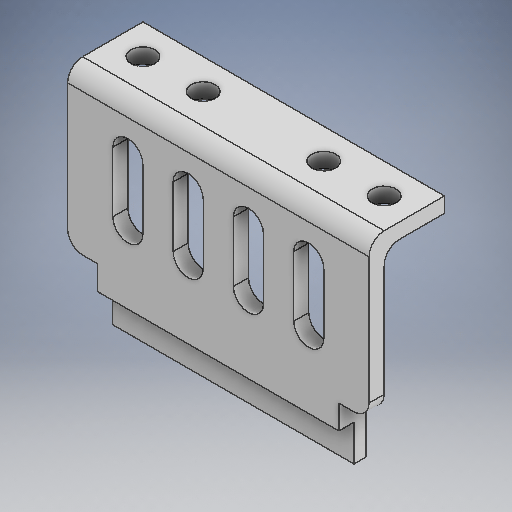
# Autodesk Inventor part: lateral_panel_1
Saved by Autodesk Inventor 2026.1 (Build 301233000, 233)
## iProperties
Created: 2025-12-05
Part Number: lateral_panel_1
Material: Generic
Document SubType Name: Modeling
Designer: emanuel
Density: 1 g/cm^3
Appearance: Default
Author: emanuel
Autodesk Inventor part; units mm, degrees
ref_plane "YZ Plane" through (0, 0, 0) normal (1, 0, 0) x (0, 1, 0)
ref_plane "XZ Plane" through (0, 0, 0) normal (0, 1, 0) x (-1, 0, 0)
ref_plane "XY Plane" through (0, 0, 0) normal (0, 0, 1) x (1, 0, 0)
sketch "Sketch1" plane through (0, 0, 0) normal (1, 0, 0) x (0, 1, 0)
  line L0 (0, 0) -> (30, 0)
  line L1 (30, 0) -> (0, 0)
  line L2 (0, 0) -> (0, -2.5)
  line L3 (0, -2.5) -> (30, -2.5)
  line L4 (30, -2.5) -> (30, 0)
  line L5 (30, -2.5) -> (27.5, -2.5)
  line L6 (27.5, -2.5) -> (27.5, -12.5)
  line L7 (27.5, -12.5) -> (30, -12.5)
  line L8 (30, -12.5) -> (30, -2.5)
  line L9 (0, -2.5) -> (2, -2.5)
  line L10 (2, -2.5) -> (2, -4.5)
  line L11 (2, -4.5) -> (0, -4.5)
  line L12 (0, -4.5) -> (0, -2.5)
  line L13 (0, -2.5) -> (-6, -2.5)
  line L14 (-6, -2.5) -> (-6, -4.5)
  line L15 (-6, -4.5) -> (0, -4.5)
  line L16 (0, -4.5) -> (0, -2.5)
  dimension "d0" = 30
  dimension "d1" = 2.5
  dimension "d2" = 2.5
  dimension "d3" = 10
  dimension "d4" = 2
  dimension "d5" = 2
  dimension "d6" = 6
  constraints: 34 end point, 8 parallel, 5 horizontal, 4 perpendicular, 1 point on line
  measures "d0" distance of L0.start L0.end
  measures "d1" distance of L2.end L1.end
  measures "d2" distance of L7.end L6.end
  measures "d3" distance of L6.end L5.end
  measures "d4" distance of L10.end L11.end
  measures "d5" distance of L9.end L10.end
  measures "d6" distance of L15.end L14.end
extrude "Extrusion1" add sketch "Sketch1" along normal blind 50
sketch "Sketch2" plane through (0, 30, 0) normal (0, 1, 0) x (1, 0, 0)
  line L0 (50, 12.5) -> (50, 0) projected
  line L1 (50, 12.5) -> (45, 12.5)
  line L2 (45, 12.5) -> (45, 7.5)
  line L3 (45, 7.5) -> (50, 7.5)
  line L4 (50, 7.5) -> (50, 12.5)
  line L5 (45, 7.5) -> (35, 7.5)
  line L6 (0, 12.5) -> (50, 12.5) projected
  line L7 (0, 12.5) -> (5, 12.5)
  line L8 (5, 12.5) -> (5, 7.5)
  line L9 (5, 7.5) -> (0, 7.5)
  line L10 (0, 7.5) -> (0, 12.5)
  circle A0 centre (5, 7.5) radius 2
  circle A1 centre (35, 7.5) radius 2
  circle A2 centre (45, 7.5) radius 2
  line L11 (5, 7.5) -> (15, 7.5)
  circle A3 centre (15, 7.5) radius 2
  point P0 (0, 0)
  dimension "d9" = 5
  dimension "d10" = 5
  dimension "d11" = 10
  dimension "d12" = 5
  dimension "d13" = 5
  dimension "d14" = 4
  dimension "d15" = 4
  dimension "d16" = 4
  dimension "d19" = 10
  dimension "d20" = 4
  constraints: 20 end point, 4 centre point, 4 coincident, 4 horizontal, 4 parallel, 2 perpendicular
  measures "d9" distance of L3.end L2.end
  measures "d10" distance of L2.end L1.end
  measures "d11" distance of L2.end L5.end
  measures "d12" distance of L8.end L9.end
  measures "d13" distance of L7.end L8.end
  measures "d14" diameter of A0
  measures "d15" diameter of A1
  measures "d16" diameter of A2
  measures "d19" distance of L11.start L11.end
  measures "d20" diameter of A3
extrude "Extrusion2" cut sketch "Sketch2" against normal blind 30 contours A1 | A3 | A2 L5 L3 | L3 L2 A2 | L2 L5 A2 | A0 L11 L8 | L8 L9 A0 | L11 A0 L9
sketch "Sketch3" plane through (0, 0, 0) normal (0, 0, 1) x (1, 0, 0)
  line L0 (0, -6) -> (0, 2) projected
  line L1 (0, -6) -> (5, -6)
  line L2 (5, -6) -> (5, 4)
  line L3 (5, 4) -> (0, 4)
  line L4 (0, 4) -> (0, -6)
  line L5 (45, -6) -> (40, -6)
  line L6 (40, -6) -> (40, 4)
  line L7 (40, 4) -> (45, 4)
  line L8 (45, 4) -> (45, -6)
  line L9 (50, -6) -> (50, 2) projected
  line L10 (50, -6) -> (45, -6)
  line L11 (45, -6) -> (45, 4)
  line L12 (45, 4) -> (50, 4)
  line L13 (50, 4) -> (50, -6)
  point P0 (0, 0)
  point P1 (0, 2)
  dimension "d21" = 5
  dimension "d22" = 10
  dimension "d23" = 5
  dimension "d24" = 10
  constraints: 24 end point, 6 parallel, 3 horizontal, 3 perpendicular, 1 point on line
  measures "d21" distance of L3.end L2.end
  measures "d22" distance of L2.end L1.end
  measures "d23" distance of L6.end L7.end
  measures "d24" distance of L5.end L6.end
extrude "Extrusion3" cut sketch "Sketch3" against normal blind 50 contours L0 L4 L3 L2 L1 | L8 L12 L13 L9 L10
sketch "Sketch4" plane through (0, 30, 0) normal (0, 0, 1) x (1, 0, 0)
  line L0 (0, 0) -> (0, -26) projected
  line L1 (0, -13) -> (50, -13)
  line L2 (50, -26) -> (50, -2.5) projected
  line L3 (0, -13) -> (10, -13)
  line L4 (10, -13) -> (20, -13)
  line L5 (20, -13) -> (30, -13)
  line L6 (30, -13) -> (40, -13)
  line L7 (40, -13) -> (50, -13)
  line L8 (7.5, -20.5) -> (12.5, -20.5)
  line L9 (12.5, -20.5) -> (12.5, -5.5)
  line L10 (12.5, -5.5) -> (7.5, -5.5)
  line L11 (7.5, -5.5) -> (7.5, -20.5)
  line L12 (7.5, -20.5) -> (12.5, -5.5) construction
  line L13 (12.5, -20.5) -> (7.5, -5.5) construction
  line L14 (17.5, -20.5) -> (22.5, -20.5)
  line L15 (22.5, -20.5) -> (22.5, -5.5)
  line L16 (22.5, -5.5) -> (17.5, -5.5)
  line L17 (17.5, -5.5) -> (17.5, -20.5)
  line L18 (17.5, -20.5) -> (22.5, -5.5) construction
  line L19 (22.5, -20.5) -> (17.5, -5.5) construction
  line L20 (27.5, -20.5) -> (32.5, -20.5)
  line L21 (32.5, -20.5) -> (32.5, -5.5)
  line L22 (32.5, -5.5) -> (27.5, -5.5)
  line L23 (27.5, -5.5) -> (27.5, -20.5)
  line L24 (27.5, -20.5) -> (32.5, -5.5) construction
  line L25 (32.5, -20.5) -> (27.5, -5.5) construction
  line L26 (37.5, -20.5) -> (42.5, -20.5)
  line L27 (42.5, -20.5) -> (42.5, -5.5)
  line L28 (42.5, -5.5) -> (37.5, -5.5)
  line L29 (37.5, -5.5) -> (37.5, -20.5)
  line L30 (37.5, -20.5) -> (42.5, -5.5) construction
  line L31 (42.5, -20.5) -> (37.5, -5.5) construction
  point P0 (0, -30)
  dimension "d27" = 10
  dimension "d28" = 10
  dimension "d29" = 10
  dimension "d30" = 10
  dimension "d31" = 10
  dimension "d32" = 5
  dimension "d33" = 15
  dimension "d34" = 5
  dimension "d35" = 15
  dimension "d36" = 5
  dimension "d37" = 15
  dimension "d38" = 5
  dimension "d39" = 15
  constraints: 60 end point, 9 equal length, 9 midpoint, 5 horizontal, 5 point on line, 4 perpendicular
  measures "d27" distance of L1.start L3.end
  measures "d28" distance of L3.end L4.end
  measures "d29" distance of L4.end L5.end
  measures "d30" distance of L5.end L6.end
  measures "d31" distance of L6.end L1.end
  measures "d32" distance of L10.end L9.end
  measures "d33" distance of L9.end L8.end
  measures "d34" distance of L16.end L15.end
  measures "d35" distance of L15.end L14.end
  measures "d36" distance of L22.end L21.end
  measures "d37" distance of L21.end L20.end
  measures "d38" distance of L28.end L27.end
  measures "d39" distance of L27.end L26.end
extrude "Extrusion4" cut sketch "Sketch4" against normal blind 50
fillet "Fillet1" radius 2.5 16 edges at (7.5, 9.5, -1.25) (12.5, 9.5, -1.25) (7.5, 24.5, -1.25) (12.5, 24.5, -1.25) (17.5, 24.5, -1.25) (22.5, 24.5, -1.25) (17.5, 9.5, -1.25) (22.5, 9.5, -1.25) (27.5, 9.5, -1.25) (27.5, 24.5, -1.25) (32.5, 24.5, -1.25) (32.5, 9.5, -1.25) (37.5, 9.5, -1.25) (37.5, 24.5, -1.25) (42.5, 24.5, -1.25) (42.5, 9.5, -1.25)
fillet "Fillet2" radius 2.5 4 edges at (25, 30, 0) (25, 27.5, -2.5) (50, 4, -1.25) (0, 4, -1.25)
body "Solid1"
